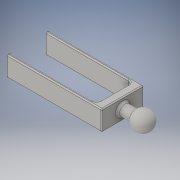
# Autodesk Inventor part: 10x20-sample-drawer-V1
Saved by Autodesk Inventor 2016 (Build 200138000, 138)
## iProperties
Created: 2018-03-02
Part Number: 10x20-sample-drawer-V1
Material: Generic
Document SubType Name: Modeling
Designer: voigt
Density: 1 g/cm^3
Appearance: Default
Author: voigt
Autodesk Inventor part; units mm, degrees
ref_plane "YZ Plane" through (0, 0, 0) normal (1, 0, 0) x (0, 1, 0)
ref_plane "XZ Plane" through (0, 0, 0) normal (0, 1, 0) x (-1, 0, 0)
ref_plane "XY Plane" through (0, 0, 0) normal (0, 0, 1) x (1, 0, 0)
sketch "Sketch1" plane through (0, 0, 0) normal (0, 0, 1) x (1, 0, 0)
  line L0 (-9, 0) -> (54, 0) construction
  line L1 (0, -13.86) -> (0, 13.86) construction
  line L2 (0, 8.5) -> (41, 8.5)
  line L3 (41, 8.5) -> (41, -8.5)
  line L4 (41, -8.5) -> (0, -8.5)
  line L5 (0, -9.9) -> (45, -9.9)
  line L6 (45, -9.9) -> (45, 9.9)
  line L7 (45, 9.9) -> (0, 9.9)
  line L8 (0, 8.5) -> (0, 9.9)
  line L9 (0, -8.5) -> (0, -9.9)
  point P0 (0, 0)
  dimension "d0" = 17
  dimension "d1" = 19.8
  dimension "d2" = 45
  dimension "d3" = 4
  constraints: 16 end point, 5 perpendicular, 4 point on line, 2 horizontal, 1 collinear, 2 other
  measures "d0" distance between parallel lines of L4 L2
  measures "d1" distance between parallel lines of L5 L7
  measures "d2" distance between parallel lines of L6 L1
  measures "d3" distance between parallel lines of L6 L3
extrude "Extrusion1" add sketch "Sketch1" along normal blind 9.5
sketch "Sketch2" plane through (45, -9.9, 0) normal (1, 0, 0) x (0, 0, -1)
  line L0 (0, 0) -> (0, 19.8) construction
  line L1 (0, 19.8) -> (-9.5, 19.8) construction
  line L2 (-9.5, 0) -> (-9.5, 19.8) construction
  line L3 (0, 0) -> (-9.5, 0) construction
  line L4 (-9.5, 0) -> (-9.5, 19.8) construction
  line L5 (-9.5, 9.9) -> (0, 9.9) construction
  line L6 (0, 0) -> (-9.5, 0) construction
  line L7 (-4.75, 0) -> (-4.75, 19.8) construction
  circle A0 centre (-4.75, 9.9) radius 2.5
  dimension "d6" = 5
  constraints: 4 end point, 4 midpoint, 1 centre point, 1 horizontal
  measures "d6" diameter of A0
extrude "Extrusion2" add sketch "Sketch2" along normal blind 9.5
ref_plane "Work Plane1" through (0, 0, 0) normal (0, -1, 0) x (1, 0, 0)
sketch "Sketch3" plane through (0, 0, 0) normal (0, -1, 0) x (1, 0, 0)
  line L0 (54.5, 2.25) -> (54.5, 7.25) construction
  line L1 (-11.7, 4.75) -> (70.2, 4.75) construction
  line L2 (54.5, 2.25) -> (54.5, 7.25) construction
  line L3 (45, 7.25) -> (45, 2.25) construction
  arc A0 (50, 4.75) -> (59, 4.75) centre (54.5, 4.75) ccw
  line L4 (59, 4.75) -> (50, 4.75)
  point P0 (0, 0)
  dimension "d9" = 4.5
  constraints: 2 end point, 2 point on circle, 1 centre point, 1 collinear, 1 midpoint, 1 point on line
  measures "d9" radius of A0
revolve "Revolution1" add sketch "Sketch3" angle 360 about axis through (45, 0, 4.75) along (1, 0, 0)
fillet "Fillet1" radius 1 1 edges at (45, 0, 7.25)
fillet "Fillet2" radius 2 2 edges at (41, -8.5, 4.75) (41, 8.5, 4.75)
fillet "Fillet3" radius 0.5 26 edges at (22.5, 9.9, 9.5) (40.4142, 7.9142, 9.5) (41, 0, 9.5) (40.4142, -7.9142, 9.5) (19.5, -8.5, 9.5) (19.5, 8.5, 9.5) (40.4142, 7.9142, 0) (41, 0, 0) (40.4142, -7.9142, 0) (19.5, -8.5, 0) (19.5, 8.5, 0) (0, 9.2, 0) (0, 9.2, 9.5) (0, -9.2, 9.5) (0, -9.2, 0) (0, -9.9, 4.75) (0, -8.5, 4.75) (22.5, -9.9, 9.5) (22.5, -9.9, 0) (0, 9.9, 4.75) (0, 8.5, 4.75) (45, 9.9, 4.75) (45, 0, 9.5) (45, -9.9, 4.75) (45, 0, 0) (22.5, 9.9, 0)
body "Solid1"
